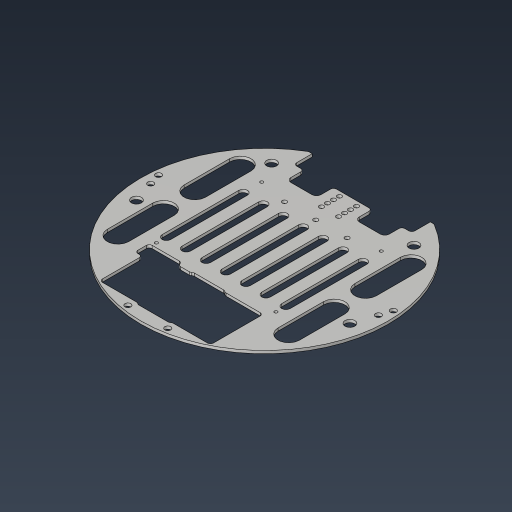
# Autodesk Inventor part: Mittelplatte
Saved by Autodesk Inventor 2023.1 (Build 271208000, 208)
## iProperties
Part Number: Mittelplatte
Material: Aluminium 6061
Document SubType Name: Modeling
Designer: rYan
Density: 2.7 g/cm^3
Appearance: Aluminium - flach
Mass: 70.3039 g
Surface Area: 310.065 cm^2
Volume: 26.0385 cm^3
Author: rYan
Autodesk Inventor part; units mm, degrees
ref_plane "YZ Plane" through (0, 0, 0) normal (1, 0, 0) x (0, 1, 0)
ref_plane "XZ Plane" through (0, 0, 0) normal (0, 1, 0) x (-1, 0, 0)
ref_plane "XY Plane" through (0, 0, 0) normal (0, 0, 1) x (1, 0, 0)
sketch "Skizze1" plane through (0, 0, 0) normal (0, 0, 1) x (1, 0, 0)
  arc A0 (-44.0908, 75) -> (44.0908, 75) centre (0, 0) ccw
  line L0 (41.5, 75) -> (41.5, 62)
  line L1 (41.5, 62) -> (-41.5, 62)
  line L2 (-41.5, 62) -> (-41.5, 75)
  line L3 (-44.0908, 75) -> (-41.5, 75)
  line L4 (41.5, 75) -> (44.0908, 75)
  line L5 (0, 107.4) -> (0, -119.4) projected
  line L6 (-121.8, 0) -> (121.8, 0) projected
  dimension "d0" = 174
  dimension "d17" = 75
  dimension "d18" = 83
  dimension "d19" = 62
  constraints: 10 end point, 2 horizontal, 2 point on circle, 1 centre point, 1 coincident, 1 parallel, 2 other
  measures "d0" diameter of A0
  measures "d17" distance between parallel lines of L6 L3
  measures "d18" distance of L0.end L1.end
  measures "d19" distance between parallel lines of L6 L1
extrude "Extrusion1" add sketch "Skizze1" along normal blind 2
sketch "Skizze2" plane through (0, 0, 0) normal (0, 0, 1) x (1, 0, 0)
  line L0 (0, 51.2) -> (0, -104.2) projected
  line L1 (-96, 0) -> (16, 0) projected
  point P0 (0, 0)
  point P1 (-82.5, 8)
  point P2 (-77, -29)
  point P3 (-14, -82)
  point P4 (-80, 0)
  dimension "d4" = 8
  dimension "d5" = 82.5
  dimension "d6" = 29
  dimension "d7" = 77
  dimension "d8" = 14
  dimension "d9" = 82
  dimension "d87" = 80
  constraints: 1 point on line
  measures "d4" distance from line of point (-82.5, 8) L1
  measures "d5" distance from line of L0 point (-82.5, 8)
  measures "d6" distance from line of point (-77, -29) L1
  measures "d7" distance from line of L0 point (-77, -29)
  measures "d8" distance from line of point (-14, -82) L0
  measures "d9" distance from line of L1 point (-14, -82)
  measures "d87" distance from line of L0 point (-80, 0)
hole "Bohrung1" at (-82.5, 8, 0) at (-14, -82, 0) at (-80, 0, 0) direction (0, 0, 1) diameter 4.2 end through all
sketch "Skizze7" plane through (0, 0, 2) normal (0, 0, 1) x (1, 0, 0)
  line L0 (-60, 11) -> (-60, 43) construction
  line L1 (-52.5, 11) -> (-52.5, 43)
  line L2 (-67.5, 43) -> (-67.5, 11)
  arc A0 (-67.5, 11) -> (-52.5, 11) centre (-60, 11) ccw
  arc A1 (-52.5, 43) -> (-67.5, 43) centre (-60, 43) ccw
  line L3 (-60, -11) -> (-60, -43) construction
  line L4 (-67.5, -11) -> (-67.5, -43)
  line L5 (-52.5, -43) -> (-52.5, -11)
  arc A2 (-52.5, -11) -> (-67.5, -11) centre (-60, -11) ccw
  arc A3 (-67.5, -43) -> (-52.5, -43) centre (-60, -43) ccw
  line L6 (0, 107.4) -> (0, -119.4) projected
  line L7 (-121.8, 0) -> (121.8, 0) projected
  point P0 (0, 0)
  point P1 (-60, 27)
  point P2 (-60, -27)
  dimension "d51" = 32
  dimension "d52" = 32
  dimension "d53" = 27
  dimension "d54" = 27
  dimension "d55" = 60
  dimension "d56" = 15
  dimension "d57" = 15
  dimension "d175" = 67.5
  dimension "d176" = 11
  dimension "d177" = 11
  constraints: 16 end point, 8 point on circle, 8 tangent, 4 centre point, 2 midpoint, 2 parallel, 2 point on line, 1 vertical
  measures "d51" distance of L0.start L0.end
  measures "d52" distance of L3.start L3.end
  measures "d53" distance from line of point (-60, 27) L7
  measures "d54" distance from line of L7 point (-60, -27)
  measures "d55" distance between parallel lines of L6 L0
  measures "d56" distance between parallel lines of L2 L1
  measures "d57" distance between parallel lines of L4 L5
  measures "d175" distance between parallel lines of L6 L4
  measures "d176" distance from line of L7 L4.start
  measures "d177" distance from line of L7 L2.end
extrude "Extrusion5" cut sketch "Skizze7" against normal through all
sketch "Skizze8" plane through (0, 0, 2) normal (0, 0, 1) x (1, 0, 0)
  line L0 (-34.5, 62) -> (-34.5, 53)
  line L1 (-13.5, 53) -> (-13.5, 62)
  arc A0 (-34.5, 53) -> (-31.5, 50) centre (-31.5, 53) ccw
  line L2 (41.5, 62) -> (-41.5, 62) projected
  line L3 (0, 107.4) -> (0, -119.4) projected
  line L4 (-31.5, 50) -> (-16.5, 50)
  arc A1 (-16.5, 50) -> (-13.5, 53) centre (-16.5, 53) ccw
  line L5 (-34.5, 62) -> (-13.5, 62)
  line L6 (-24, 50) -> (-24, 62) construction
  point P0 (0, 0)
  dimension "d60" = 21
  dimension "d131" = 3
  dimension "d133" = 24
  dimension "d134" = 12
  constraints: 10 end point, 4 point on circle, 4 tangent, 2 centre point, 2 midpoint, 2 vertical, 1 collinear, 1 horizontal, 1 parallel, 1 perpendicular
  measures "d60" distance between parallel lines of L0 L1
  measures "d131" radius of A1
  measures "d133" distance between parallel lines of L3 L6
  measures "d134" distance between parallel lines of L2 L4
extrude "Extrusion6" cut sketch "Skizze8" against normal through all
sketch "Skizze11" plane through (0, 0, 2) normal (0, 0, 1) x (1, 0, 0)
  line L0 (0, 107.4) -> (0, -119.4) projected
  line L1 (-121.8, 0) -> (121.8, 0) projected
  point P0 (0, 0)
  point P1 (-50, 55)
  point P2 (-75, -15)
  dimension "d90" = 15
  dimension "d135" = 75
  dimension "d136" = 55
  dimension "d137" = 50
  measures "d90" distance from line of point (-75, -15) L1
  measures "d135" distance from line of L0 point (-75, -15)
  measures "d136" distance from line of point (-50, 55) L1
  measures "d137" distance from line of L0 point (-50, 55)
hole "Bohrung5" at (-50, 55, 2) at (-75, -15, 2) direction (0, 0, -1) diameter 7 end through all
sketch "Skizze14" plane through (0, 0, 2) normal (0, 0, 1) x (1, 0, 0)
  line L0 (0, 107.4) -> (0, -119.4) projected
  line L1 (-121.8, 0) -> (121.8, 0) projected
  point P0 (0, 0)
  point P1 (-42, 40)
  point P2 (-42, -34)
  dimension "d120" = 42
  dimension "d121" = 40
  dimension "d122" = 42
  dimension "d123" = 34
  measures "d120" distance from line of L0 point (-42, 40)
  measures "d121" distance from line of point (-42, 40) L1
  measures "d122" distance from line of point (-42, -34) L0
  measures "d123" distance from line of point (-42, -34) L1
hole "Powerboard" at (-42, 40, 2) at (-42, -34, 2) direction (0, 0, -1) diameter 2.2 end through all
mirror "Spiegeln2" about plane through (0, 0, 0) normal (1, 0, 0) of "Extrusion5", "Bohrung1", "Extrusion6", "Bohrung5", "Powerboard"
sketch "Skizze5" plane through (0, 0, 2) normal (0, 0, 1) x (1, 0, 0)
  line L0 (39, -77) -> (39, -40)
  line L1 (-39, -47) -> (-39, -77)
  line L2 (0, 107.4) -> (0, -119.4) projected
  line L3 (-21, -37) -> (-21, -40)
  line L4 (-39, -37) -> (-44, -37)
  line L5 (-44, -37) -> (-44, -47)
  line L6 (-44, -47) -> (-39, -47)
  line L7 (-21, -37) -> (-39, -37)
  line L8 (12, -40) -> (12, -39)
  line L9 (12, -39) -> (-12, -39)
  line L10 (-12, -39) -> (-12, -40)
  line L11 (12, -77) -> (12, -78)
  line L12 (12, -78) -> (-12, -78)
  line L13 (-12, -78) -> (-12, -77)
  line L14 (-21, -40) -> (-12, -40)
  line L15 (12, -40) -> (39, -40)
  line L16 (-39, -77) -> (-12, -77)
  line L17 (12, -77) -> (39, -77)
  point P0 (0, 0)
  dimension "d139" = 37
  dimension "d140" = 78
  dimension "d141" = 37
  dimension "d142" = 18
  dimension "d143" = 10
  dimension "d144" = 5
  dimension "d145" = 1
  dimension "d146" = 1
  dimension "d147" = 24
  dimension "d148" = 30
  constraints: 34 end point, 6 perpendicular, 5 horizontal, 5 parallel, 2 collinear, 2 point on line, 1 vertical, 3 other
  measures "d139" distance from line of point (0, 0) L7
  measures "d140" distance between parallel lines of L0 L1
  measures "d141" distance of L0.start L0.end
  measures "d142" distance between parallel lines of L3 L1
  measures "d143" distance of L4.end L5.end
  measures "d144" distance of L5.end L1.start
  measures "d145" distance of L9.end L10.end
  measures "d146" distance of L12.end L13.end
  measures "d147" distance of L8.end L9.end
  measures "d148" distance of L1.start L1.end
extrude "Extrusion4" cut sketch "Skizze5" against normal through all
fillet "Rundung1" radius 2 8 edges at (39, -40, 1) (39, -77, 1) (-39, -77, 1) (-21, -40, 1) (-21, -37, 1) (-44, -37, 1) (-44, -47, 1) (-39, -47, 1)
sketch "Skizze6" plane through (0, 0, 2) normal (0, 0, 1) x (1, 0, 0)
  line L0 (0, 107.4) -> (0, -119.4) projected
  line L1 (-121.8, 0) -> (121.8, 0) projected
  line L2 (-22, 36) -> (22, 36) construction
  point P0 (0, 0)
  point P1 (0, 36)
  dimension "d42" = 22
  dimension "d43" = 36
  constraints: 2 coincident, 2 end point, 1 horizontal, 1 midpoint, 1 point on line
  measures "d42" distance of point (0, 36) point (-22, 36)
  measures "d43" distance between parallel lines of L1 L2
hole "Bohrung2" at (0, 36, 2) at (22, 36, 2) at (-22, 36, 2) direction (0, 0, -1) diameter 3.2 end through all
sketch "Skizze9" plane through (0, 0, 2) normal (0, 0, 1) x (1, 0, 0)
  line L0 (0, 107.4) -> (0, -119.4) projected
  line L1 (-121.8, 0) -> (121.8, 0) projected
  line L2 (-6, 46) -> (6, 46) construction
  point P0 (0, 0)
  dimension "d65" = 12
  dimension "d66" = 46
  constraints: 2 coincident, 2 end point, 1 horizontal, 1 symmetric about line
  measures "d65" distance of L2.start L2.end
  measures "d66" distance between parallel lines of L1 L2
hole "Bohrung3" at (-6, 46, 2) at (6, 46, 2) direction (0, 0, -1) diameter 3.2 end through all
pattern_linear "Rechteckige Anordnung1" count 4 spacing 4.2 along (0, 1, 0) of "Bohrung3"
fillet "Rundung2" radius 2 8 edges at (-12, -40, 1) (-12, -39, 1) (12, -40, 1) (12, -39, 1) (-12, -77, 1) (-12, -78, 1) (12, -77, 1) (12, -78, 1)
sketch "Skizze15" plane through (0, 0, 2) normal (0, 0, 1) x (1, 0, 0)
  line L0 (0, 27) -> (0, -27) construction
  line L1 (-3, 27) -> (-3, -27)
  line L2 (3, -27) -> (3, 27)
  arc A0 (3, 27) -> (-3, 27) centre (0, 27) ccw
  arc A1 (-3, -27) -> (3, -27) centre (0, -27) ccw
  point P0 (0, 0)
  point P1 (0, 0)
  dimension "d150" = 6
  dimension "d151" = 54
  constraints: 8 end point, 4 point on circle, 4 tangent, 2 centre point, 2 midpoint, 1 coincident, 1 parallel, 1 vertical
  measures "d150" distance between parallel lines of L1 L2
  measures "d151" distance of L0.start L0.end
extrude "Extrusion7" cut sketch "Skizze15" against normal through all
pattern_linear "Rechteckige Anordnung2" count 7 spacing 14 along (1, 0, 0) of "Extrusion7" first direction both ways yes
sketch "Skizze16" plane through (0, 0, 2) normal (0, 0, 1) x (1, 0, 0)
  line L0 (0, 107.4) -> (0, -119.4) projected
  line L1 (-121.8, 0) -> (121.8, 0) projected
  line L2 (-48, -60) -> (48, -60) construction
  line L3 (-48, 65) -> (48, 65) construction
  point P0 (0, 0)
  point P1 (0, -35)
  dimension "d158" = 96
  dimension "d159" = 60
  dimension "d160" = 35
  dimension "d161" = 65
  dimension "d162" = 96
  constraints: 4 coincident, 4 end point, 2 horizontal, 2 symmetric about line, 1 point on line
  measures "d158" distance of L2.start L2.end
  measures "d159" distance between parallel lines of L1 L2
  measures "d160" distance from line of point (0, -35) L1
  measures "d161" distance between parallel lines of L3 L1
  measures "d162" distance of L3.start L3.end
hole "Bohrung9" [suppressed]
sketch "Fertigung" plane through (0, 0, 0) normal (0, 0, 1) x (1, 0, 0)
  arc A0 (45, 27) -> (39, 27) centre (42, 27) ccw projected
  line L0 (39, 27) -> (39, -27) projected
  arc A1 (39, -27) -> (45, -27) centre (42, -27) ccw projected
  line L1 (45, -27) -> (45, 27) projected
  arc A2 (31, 27) -> (25, 27) centre (28, 27) ccw projected
  line L2 (25, 27) -> (25, -27) projected
  arc A3 (25, -27) -> (31, -27) centre (28, -27) ccw projected
  line L3 (31, -27) -> (31, 27) projected
  arc A4 (17, 27) -> (11, 27) centre (14, 27) ccw projected
  line L4 (11, 27) -> (11, -27) projected
  arc A5 (11, -27) -> (17, -27) centre (14, -27) ccw projected
  line L5 (17, -27) -> (17, 27) projected
  arc A6 (-11, 27) -> (-17, 27) centre (-14, 27) ccw projected
  line L6 (-17, 27) -> (-17, -27) projected
  arc A7 (-17, -27) -> (-11, -27) centre (-14, -27) ccw projected
  line L7 (-11, -27) -> (-11, 27) projected
  arc A8 (-25, 27) -> (-31, 27) centre (-28, 27) ccw projected
  line L8 (-31, 27) -> (-31, -27) projected
  arc A9 (-31, -27) -> (-25, -27) centre (-28, -27) ccw projected
  line L9 (-25, -27) -> (-25, 27) projected
  arc A10 (-39, 27) -> (-45, 27) centre (-42, 27) ccw projected
  line L10 (-45, 27) -> (-45, -27) projected
  arc A11 (-45, -27) -> (-39, -27) centre (-42, -27) ccw projected
  line L11 (-39, -27) -> (-39, 27) projected
  arc A12 (-3, -27) -> (3, -27) centre (0, -27) ccw projected
  line L12 (3, -27) -> (3, 27) projected
  arc A13 (3, 27) -> (-3, 27) centre (0, 27) ccw projected
  line L13 (-3, 27) -> (-3, -27) projected
  arc A14 (12.9137, -77) -> (11.5908, -77.5) centre (12.9137, -79) ccw projected
  line L14 (12.9137, -77) -> (37, -77) projected
  arc A15 (37, -77) -> (39, -75) centre (37, -75) ccw projected
  line L15 (39, -75) -> (39, -42) projected
  arc A16 (39, -42) -> (37, -40) centre (37, -42) ccw projected
  line L16 (37, -40) -> (12.9137, -40) projected
  arc A17 (11.5908, -39.5) -> (12.9137, -40) centre (12.9137, -38) ccw projected
  arc A18 (11.5908, -39.5) -> (10.2679, -39) centre (10.2679, -41) ccw projected
  line L17 (10.2679, -39) -> (-10.2679, -39) projected
  arc A19 (-10.2679, -39) -> (-11.5908, -39.5) centre (-10.2679, -41) ccw projected
  arc A20 (-12.9137, -40) -> (-11.5908, -39.5) centre (-12.9137, -38) ccw projected
  line L18 (-12.9137, -40) -> (-19, -40) projected
  arc A21 (-20.9365, -38.5) -> (-19, -40) centre (-19, -38) ccw projected
  arc A22 (-20.9365, -38.5) -> (-22.873, -37) centre (-22.873, -39) ccw projected
  line L19 (-22.873, -37) -> (-42, -37) projected
  arc A23 (-42, -37) -> (-44, -39) centre (-42, -39) ccw projected
  line L20 (-44, -39) -> (-44, -45) projected
  arc A24 (-44, -45) -> (-42, -47) centre (-42, -45) ccw projected
  line L21 (-42, -47) -> (-41, -47) projected
  arc A25 (-39, -49) -> (-41, -47) centre (-41, -49) ccw projected
  line L22 (-39, -49) -> (-39, -75) projected
  arc A26 (-39, -75) -> (-37, -77) centre (-37, -75) ccw projected
  line L23 (-37, -77) -> (-12.9137, -77) projected
  arc A27 (-11.5908, -77.5) -> (-12.9137, -77) centre (-12.9137, -79) ccw projected
  arc A28 (-11.5908, -77.5) -> (-10.2679, -78) centre (-10.2679, -76) ccw projected
  line L24 (-10.2679, -78) -> (10.2679, -78) projected
  arc A29 (10.2679, -78) -> (11.5908, -77.5) centre (10.2679, -76) ccw projected
  circle A30 centre (-6, 58.6) radius 1.6 projected
  circle A31 centre (6, 58.6) radius 1.6 projected
  circle A32 centre (-6, 54.4) radius 1.6 projected
  circle A33 centre (6, 54.4) radius 1.6 projected
  circle A34 centre (-6, 50.2) radius 1.6 projected
  circle A35 centre (6, 50.2) radius 1.6 projected
  circle A36 centre (-6, 46) radius 1.6 projected
  circle A37 centre (6, 46) radius 1.6 projected
  circle A38 centre (22, 36) radius 1.6 projected
  circle A39 centre (0, 36) radius 1.6 projected
  circle A40 centre (-22, 36) radius 1.6 projected
  circle A41 centre (50, 55) radius 3.5 projected
  circle A42 centre (75, -15) radius 3.5 projected
  arc A43 (52.5, 11) -> (67.5, 11) centre (60, 11) ccw projected
  line L25 (67.5, 11) -> (67.5, 43) projected
  arc A44 (67.5, 43) -> (52.5, 43) centre (60, 43) ccw projected
  line L26 (52.5, 43) -> (52.5, 11) projected
  line L27 (52.5, -11) -> (52.5, -43) projected
  arc A45 (52.5, -43) -> (67.5, -43) centre (60, -43) ccw projected
  line L28 (67.5, -43) -> (67.5, -11) projected
  arc A46 (67.5, -11) -> (52.5, -11) centre (60, -11) ccw projected
  circle A47 centre (14, -82) radius 2.1 projected
  circle A48 centre (80, 0) radius 2.1 projected
  circle A49 centre (82.5, 8) radius 2.1 projected
  circle A50 centre (42, -34) radius 1.1 projected
  circle A51 centre (42, 40) radius 1.1 projected
  circle A52 centre (-42, 40) radius 1.1 projected
  circle A53 centre (-42, -34) radius 1.1 projected
  circle A54 centre (-50, 55) radius 3.5 projected
  circle A55 centre (-75, -15) radius 3.5 projected
  line L29 (13.5, 62) -> (13.5, 53) projected
  arc A56 (13.5, 53) -> (16.5, 50) centre (16.5, 53) ccw projected
  line L30 (16.5, 50) -> (31.5, 50) projected
  arc A57 (31.5, 50) -> (34.5, 53) centre (31.5, 53) ccw projected
  line L31 (34.5, 53) -> (34.5, 62) projected
  line L32 (41.5, 62) -> (34.5, 62) projected
  line L33 (41.5, 75) -> (41.5, 62) projected
  line L34 (44.0908, 75) -> (41.5, 75) projected
  arc A58 (-44.0908, 75) -> (44.0908, 75) centre (0, 0) ccw projected
  line L35 (-41.5, 75) -> (-44.0908, 75) projected
  line L36 (-41.5, 62) -> (-41.5, 75) projected
  line L37 (-34.5, 62) -> (-41.5, 62) projected
  line L38 (-34.5, 62) -> (-34.5, 53) projected
  arc A59 (-34.5, 53) -> (-31.5, 50) centre (-31.5, 53) ccw projected
  line L39 (-31.5, 50) -> (-16.5, 50) projected
  arc A60 (-16.5, 50) -> (-13.5, 53) centre (-16.5, 53) ccw projected
  line L40 (-13.5, 53) -> (-13.5, 62) projected
  line L41 (13.5, 62) -> (-13.5, 62) projected
  circle A61 centre (-80, 0) radius 2.1 projected
  circle A62 centre (-82.5, 8) radius 2.1 projected
  circle A63 centre (-14, -82) radius 2.1 projected
  arc A64 (-67.5, -43) -> (-52.5, -43) centre (-60, -43) ccw projected
  line L42 (-52.5, -43) -> (-52.5, -11) projected
  arc A65 (-52.5, -11) -> (-67.5, -11) centre (-60, -11) ccw projected
  line L43 (-67.5, -11) -> (-67.5, -43) projected
  arc A66 (-52.5, 43) -> (-67.5, 43) centre (-60, 43) ccw projected
  line L44 (-67.5, 43) -> (-67.5, 11) projected
  arc A67 (-67.5, 11) -> (-52.5, 11) centre (-60, 11) ccw projected
  line L45 (-52.5, 11) -> (-52.5, 43) projected
  line L46 (-60, 43) -> (-60, 11) construction
  line L47 (-60, -11) -> (-60, -43) construction
  line L48 (60, 43) -> (60, 11) construction
  line L49 (60, -11) -> (60, -43) construction
  line L50 (39, -42) -> (39, -75) construction
  line L51 (39, -58.5) -> (-39, -58.5) construction
  line L52 (-39, -75) -> (-39, -49) construction
  line L53 (0, 107.4) -> (0, -119.4) projected
  line L54 (-29, -50) -> (29, -50) construction
  line L55 (29, -50) -> (29, -67) construction
  line L56 (29, -67) -> (-29, -67) construction
  line L57 (-29, -67) -> (-29, -50) construction
  point P0 (-60, -27)
  point P1 (-60, 27)
  point P2 (60, 27)
  point P3 (60, -27)
  dimension "d171" = 10
  dimension "d172" = 10
  dimension "d173" = 10
  constraints: 18 end point, 12 coincident, 5 midpoint, 4 vertical, 2 parallel, 2 perpendicular, 1 horizontal, 1 point on line, 1 other
  measures "d171" distance between parallel lines of L52 L57
  measures "d172" distance between parallel lines of L16 L54
  measures "d173" distance between parallel lines of L56 L14
fillet "Rundung3" radius 2 8 edges at (41.5, 62, 1) (34.5, 62, 1) (13.5, 62, 1) (-13.5, 62, 1) (-34.5, 62, 1) (-41.5, 62, 1) (-44.0908, 75, 1) (44.0908, 75, 1)
equation "\"d52\" = d51"
